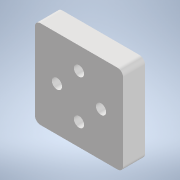
# Autodesk Inventor part: 8mmSpacer
Saved by Autodesk Inventor 2020.1 (Build 241239000, 239)
## iProperties
Created: 2019-12-07
Part Number: 8mmSpacer
Material: Generic
Document SubType Name: Modeling
Designer: alpha
Density: 1 g/cm^3
Appearance: Default
Author: alpha
Autodesk Inventor part; units mm, degrees
ref_plane "YZ Plane" through (0, 0, 0) normal (1, 0, 0) x (0, 1, 0)
ref_plane "XZ Plane" through (0, 0, 0) normal (0, 1, 0) x (-1, 0, 0)
ref_plane "XY Plane" through (0, 0, 0) normal (0, 0, 1) x (1, 0, 0)
sketch "Sketch1" plane through (0, 0, 0) normal (0, 0, 1) x (1, 0, 0)
  line L0 (0, 0) -> (32, 0)
  line L1 (32, 0) -> (32, 32)
  line L2 (32, 32) -> (0, 32)
  line L3 (0, 32) -> (0, 0)
  circle A0 centre (24, 16) radius 1.85 projected
  circle A1 centre (16, 24) radius 1.85 projected
  circle A2 centre (8, 16) radius 1.85 projected
  circle A3 centre (16, 8) radius 1.85 projected
  dimension "d0" = 32
  dimension "d1" = 32
  constraints: 8 end point, 2 parallel, 1 horizontal, 1 perpendicular
  measures "d0" distance of L2.end L1.end
  measures "d1" distance of L1.end L0.end
extrude "Extrusion1" add sketch "Sketch1" along normal blind 8
fillet "Fillet1" radius 2 4 edges at (32, 0, 4) (32, 32, 4) (0, 0, 4) (0, 32, 4)
body "Solid1"
